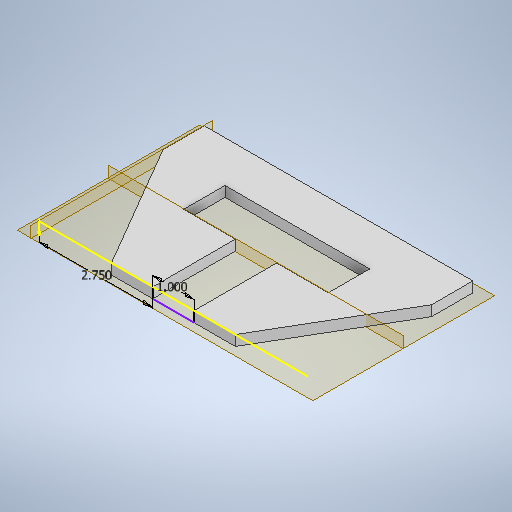
# Autodesk Inventor part: chap3ex1
Saved by Autodesk Inventor 2025.2 (Build 292293000, 293)
## iProperties
Created: 2025-02-01
Part Number: chap3ex1
Material: Generic
Document SubType Name: Modeling
Designer: Moofin
Density: 1 g/cm^3
Appearance: Default
Author: Moofin
Autodesk Inventor part; units mm, degrees
sketch "Sketch1" plane through (0, 0, 0) normal (0, 1, 0) x (-1, 0, 0)
  line L0 (0, -50.8) -> (-165.1, -50.8)
  line L1 (-165.1, -50.8) -> (-165.1, 50.8)
  line L2 (-165.1, 50.8) -> (0, 50.8)
  line L3 (0, 50.8) -> (0, -50.8)
  line L4 (0, -71.12) -> (0, 71.12) projected
  line L5 (-198.12, 0) -> (33.02, 0) projected
  point P0 (0, 0)
  dimension "d0" = 0
  dimension "d1" = 101.6
  dimension "d2" = 50.8
  dimension "d3" = 165.1
  constraints: 8 end point, 2 parallel, 1 horizontal, 1 perpendicular
  measures "d0" distance between parallel lines of L4 L3
  measures "d1" distance between parallel lines of L2 L0
  measures "d2" distance between parallel lines of L5 L0
  measures "d3" distance between parallel lines of L1 L3
extrude "Extrusion1" add sketch "Sketch1" along normal blind 6.35
chamfer "Chamfer1" distance 76.2 distance2 44.45 1 edges at (0, 3.175, 50.8) measured on face at (0, 2.1167, -16.9333)
chamfer "Chamfer2" distance 44.45 distance2 76.2 1 edges at (165.1, 3.175, 50.8) measured on face at (84.6667, 2.1167, 50.8)
sketch "Sketch2" plane through (0, 6.35, 0) normal (0, 1, 0) x (1, 0, 0)
  line L0 (38.1, 25.4) -> (127, 25.4)
  line L1 (127, 25.4) -> (127, 0)
  line L2 (127, 0) -> (38.1, 0)
  line L3 (38.1, 0) -> (38.1, 25.4)
  line L4 (165.1, 50.8) -> (0, 50.8) projected
  line L5 (0, 50.8) -> (0, 25.4) projected
  point P0 (0, 0)
  point P1 (38.1, 12.7)
  dimension "d12" = 25.4
  dimension "d13" = 25.4
  dimension "d14" = 88.9
  dimension "d15" = 38.1
  constraints: 8 end point, 2 parallel, 1 horizontal, 1 midpoint, 1 perpendicular
  measures "d12" distance of L0.end L1.end
  measures "d13" distance between parallel lines of L4 L0
  measures "d14" distance from line of L1 point (38.1, 12.7)
  measures "d15" distance between parallel lines of L5 L3
extrude "Extrusion2" cut sketch "Sketch2" against normal up to surface (6.35 mm away)
sketch "Sketch3" plane through (44.45, 0, 50.8) normal (0, 0, 1) x (1, 0, 0)
  line L0 (120.65, 6.35) -> (-44.45, 6.35) projected
  line L1 (25.4, 6.35) -> (25.4, 0)
  line L2 (25.4, 0) -> (50.8, 0)
  line L3 (50.8, 0) -> (50.8, 6.35)
  line L4 (-44.45, 7.62) -> (-44.45, -1.27) projected
  point P0 (-44.45, 0)
  dimension "d18" = 25.4
  dimension "d19" = 69.85
  constraints: 6 end point, 3 perpendicular, 2 point on line
  measures "d18" distance between parallel lines of L3 L1
  measures "d19" distance between parallel lines of L4 L1
sketch "Sketch4" plane through (127, 6.35, 0) normal (0, 0, -1) x (-1, 0, 0)
  line L0 (88.9, -6.35) -> (0, -6.35) projected
  line L1 (88.9, 0) -> (88.9, -6.35) projected
  line L2 (0, 0) -> (88.9, 0) projected
  line L3 (0, 0) -> (0, -6.35) projected
  line L4 (31.75, -6.35) -> (31.75, 0) projected
  line L5 (57.15, 0) -> (57.15, -6.35) projected
  point P0 (127, -6.35)
extrude "Extrusion3" cut sketch "Sketch4" against normal up to next contours L0 L4 L2 L5
equation "\"d2\" = 0.5 * d1"
body "Solid1"
